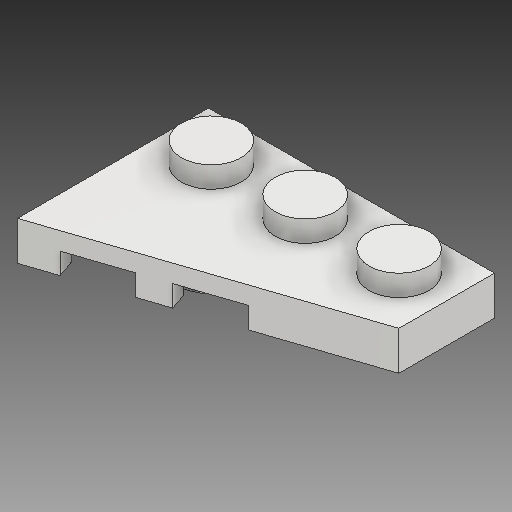
# Autodesk Inventor part: 3x1 diagonal
Saved by Autodesk Inventor 2017 (Build 210142000, 142)
## iProperties
Created: 2018-05-10
Part Number: 3x1 diagonal
Material: ABS Plastic
Document SubType Name: Modeling
Designer: 20000694
Density: 1.06 g/cm^3
Appearance: Smooth - White
Mass: 0.718798 g
Surface Area: 10.9638 cm^2
Volume: 0.678111 cm^3
Author: 20000694
Autodesk Inventor part; units mm, degrees
ref_plane "YZ Plane" through (0, 0, 0) normal (1, 0, 0) x (0, 1, 0)
ref_plane "XZ Plane" through (0, 0, 0) normal (0, 1, 0) x (-1, 0, 0)
ref_plane "XY Plane" through (0, 0, 0) normal (0, 0, 1) x (1, 0, 0)
sketch "Sketch1" plane through (0, 0, 0) normal (0, 0, 1) x (1, 0, 0)
  line L0 (0, 0) -> (0, 23.7553)
  line L1 (0, 0) -> (15.875, 0)
  line L2 (0, 23.7553) -> (7.9451, 23.7553)
  line L3 (7.9451, 23.7553) -> (15.875, 0)
  line L4 (7.9451, 23.7553) -> (31.7005, 23.7553) construction
  line L5 (0, 23.7553) -> (0, 15.8369)
  line L6 (0, 0) -> (0, 7.9184)
  dimension "d0" = 23.7553
  dimension "d1" = 15.875
  dimension "d2" = 7.9451
  dimension "d10" = 7.9185
  constraints: 14 end point, 3 horizontal, 2 point on line, 1 collinear, 1 vertical
  measures "d0" distance of L0.start L0.end
  measures "d1" distance of L0.start L1.end
  measures "d2" distance of L0.end L2.end
  measures "d10" distance of L0.end L5.end
extrude "Extrusion2" add sketch "Sketch1" along normal blind 3.236
sketch "Sketch3" plane through (0, 0, 3.236) normal (0, 0, 1) x (1, 0, 0)
  line L0 (15.875, 0) -> (7.9451, 23.7553) projected
  line L1 (0, 0) -> (15.875, 0) projected
  line L2 (7.9451, 23.7553) -> (7.9451, 0)
  line L3 (7.9451, 23.7553) -> (0, 23.7553) projected
  line L4 (0, 23.7553) -> (0, 15.8369)
  line L5 (0, 23.7553) -> (0, 0) projected
  line L6 (0, 15.8369) -> (0, 7.9184)
  circle A0 centre (3.9726, 19.7961) radius 2.4879
  dimension "d17" = 4.9759
  constraints: 6 end point, 3 point on line, 1 centre point, 1 perpendicular
  measures "d17" diameter of A0
extrude "Extrusion3" add sketch "Sketch3" along normal blind 1.7577 contours A0
pattern_linear "Rectangular Pattern2" count 3 spacing 7.7978 along (0, -1, 0) of "Extrusion3"
shell "Shell1" thickness 1.4732 removed faces 1 at (7.94, 7.9185, 0)
sketch "Sketch5" plane through (13.8301, 1.4732, 1.7628) normal (0, 0, -1) x (-1, 0, 0)
  circle A0 centre (5.9587, 6.6262) radius 2.4498
  circle A1 centre (5.9587, 6.6262) radius 3.0259
  circle A2 centre (9.8576, 2.7273) radius 2.4879 construction
  circle A3 centre (9.8576, 10.5251) radius 2.4879 construction
  line L0 (9.8576, 10.5251) -> (2.0598, 10.5251) construction
  line L1 (2.0598, 10.5251) -> (2.0598, 2.7273) construction
  line L2 (2.0598, 2.7273) -> (9.8576, 2.7273) construction
  line L3 (9.8576, 2.7273) -> (9.8576, 10.5251) construction
  line L4 (9.8576, 10.5251) -> (2.0598, 2.7273) construction
  point P0 (13.8301, -1.4732)
  dimension "d39" = 7.7978
  dimension "d40" = 7.7978
  dimension "d41" = 4.8997
  constraints: 10 end point, 2 centre point, 2 parallel, 1 coincident, 1 horizontal, 1 midpoint, 1 perpendicular, 1 tangent
  measures "d39" distance of L2.end L1.end
  measures "d40" distance of L1.end L0.end
  measures "d41" diameter of A0
extrude "Extrusion4" add sketch "Sketch5" along normal up to surface (1.7628 mm away)
pattern_linear "Rectangular Pattern3" count 2 spacing 7.7978 along (0, 1, 0) of "Extrusion4"
sketch "Sketch6" plane through (0, 0, 0) normal (0, 0, -1) x (-1, 0, 0)
  circle A0 centre (-3.9726, 4.2005) radius 2.4879 projected
  line L0 (-3.9726, 4.2005) -> (-11.7704, 4.2005) construction
  arc A1 (-12.5581, 1.8406) -> (-10.9826, 6.5604) centre (-11.7704, 4.2005) ccw
  circle A2 centre (-7.8715, 8.0994) radius 3.0259 projected
  line L1 (-10.9826, 6.5604) -> (-20.4448, 9.7191)
  line L2 (-12.5581, 1.8406) -> (-25.2023, 6.0614)
  line L3 (-25.2023, 6.0614) -> (-20.4448, 9.7191)
  line L4 (-15.875, 0) -> (-10.8097, 15.174) projected
  point P0 (0, 0)
  dimension "d42" = 7.7978
  constraints: 8 end point, 3 tangent, 2 perpendicular, 2 point on circle, 1 centre point, 1 coincident, 1 horizontal
  measures "d42" distance of L0.start L0.end
extrude "Extrusion5" cut sketch "Sketch6" against normal up to surface (1.7628 mm away) contours A1 L2 L4 L1 | L2 L3 L1 L4
sketch "Sketch7" plane through (0, 0, 0) normal (0, 0, -1) x (-1, 0, 0)
  circle A0 centre (-3.9726, 11.9983) radius 2.4879 projected
  line L0 (-3.9726, 11.9983) -> (-11.7704, 11.9983) construction
  circle A1 centre (-11.7704, 11.9983) radius 2.4879
  circle A2 centre (-7.8715, 8.0994) radius 3.0259 projected
  line L1 (-13.4141, 7.3721) -> (-10.8097, 15.174) projected
  line L2 (-11.0726, 14.3864) -> (-8.7367, 21.384)
  line L3 (-8.7367, 21.384) -> (-11.249, 21.384)
  line L4 (-11.249, 21.384) -> (-14.0474, 13.0007)
  line L5 (-25.9039, 14.0934) -> (-10.7493, 9.0346)
  line L6 (-24.9299, 19.014) -> (-10.9826, 14.3582)
  line L7 (-24.9299, 19.014) -> (-25.9039, 14.0934)
  line L8 (-10.7493, 9.0346) -> (-11.1181, 9.5974)
  line L9 (-12.0167, 6.9056) -> (-9.7949, 13.5613) projected
  point P0 (0, 0)
  dimension "d45" = 7.7978
  constraints: 16 end point, 4 point on circle, 3 perpendicular, 2 horizontal, 2 point on line, 2 tangent, 1 centre point, 1 coincident, 1 collinear, 3 other
  measures "d45" distance of L0.start L0.end
extrude "Extrusion6" cut sketch "Sketch7" against normal up to surface (1.7628 mm away) contours L1 A1 L9 | A1 L9 | L5 L9 L8 | L5 L7 L6 L4 A1 | A1 L1 | L9 L5 A1 | L4 L6 A1 | L6 L4 L3 L2 L1
body "Solid2"
